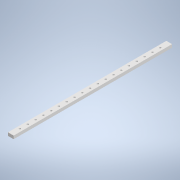
# Autodesk Inventor part: ServoArm
Saved by Autodesk Inventor 2020 (Build 240168000, 168)
## iProperties
Created: 2020-02-26
Part Number: ServoArm
Material: Generic
Document SubType Name: Modeling
Designer: shrey
Density: 1 g/cm^3
Appearance: Default
Author: shrey
Autodesk Inventor part; units mm, degrees
ref_plane "YZ Plane" through (0, 0, 0) normal (1, 0, 0) x (0, 1, 0)
ref_plane "XZ Plane" through (0, 0, 0) normal (0, 1, 0) x (-1, 0, 0)
ref_plane "XY Plane" through (0, 0, 0) normal (0, 0, 1) x (1, 0, 0)
sketch "Sketch1" plane through (0, 0, 0) normal (0, 1, 0) x (-1, 0, 0)
  line L0 (5.872, 162.6948) -> (-5.872, 162.6948)
  line L1 (-5.872, 162.6948) -> (-5.872, -162.6948)
  line L2 (-5.872, -162.6948) -> (5.872, -162.6948)
  line L3 (5.872, -162.6948) -> (5.872, 162.6948)
  line L4 (5.872, 162.6948) -> (-5.872, -162.6948) construction
  line L5 (-5.872, 162.6948) -> (5.872, -162.6948) construction
  circle A0 centre (0, 0) radius 1.85
  circle A1 centre (0, 16) radius 1.85
  circle A2 centre (0, 32) radius 1.85
  circle A3 centre (0, 48) radius 1.85
  circle A4 centre (0, 64) radius 1.85
  circle A5 centre (0, 80) radius 1.85
  circle A6 centre (0, 96) radius 1.85
  circle A7 centre (0, 112) radius 1.85
  circle A8 centre (0, 128) radius 1.85
  circle A9 centre (0, 144) radius 1.85
  circle A10 centre (0, -16) radius 1.85
  circle A11 centre (0, 0) radius 1.85
  circle A12 centre (0, 16) radius 1.85
  circle A13 centre (0, 32) radius 1.85
  circle A14 centre (0, 48) radius 1.85
  circle A15 centre (0, 64) radius 1.85
  circle A16 centre (0, 80) radius 1.85
  circle A17 centre (0, 96) radius 1.85
  circle A18 centre (0, 112) radius 1.85
  circle A19 centre (0, 128) radius 1.85
  circle A20 centre (0, -32) radius 1.85
  circle A21 centre (0, -16) radius 1.85
  circle A22 centre (0, 0) radius 1.85
  circle A23 centre (0, 16) radius 1.85
  circle A24 centre (0, 32) radius 1.85
  circle A25 centre (0, 48) radius 1.85
  circle A26 centre (0, 64) radius 1.85
  circle A27 centre (0, 80) radius 1.85
  circle A28 centre (0, 96) radius 1.85
  circle A29 centre (0, 112) radius 1.85
  circle A30 centre (0, -48) radius 1.85
  circle A31 centre (0, -32) radius 1.85
  circle A32 centre (0, -16) radius 1.85
  circle A33 centre (0, 0) radius 1.85
  circle A34 centre (0, 16) radius 1.85
  circle A35 centre (0, 32) radius 1.85
  circle A36 centre (0, 48) radius 1.85
  circle A37 centre (0, 64) radius 1.85
  circle A38 centre (0, 80) radius 1.85
  circle A39 centre (0, 96) radius 1.85
  circle A40 centre (0, -64) radius 1.85
  circle A41 centre (0, -48) radius 1.85
  circle A42 centre (0, -32) radius 1.85
  circle A43 centre (0, -16) radius 1.85
  circle A44 centre (0, 0) radius 1.85
  circle A45 centre (0, 16) radius 1.85
  circle A46 centre (0, 32) radius 1.85
  circle A47 centre (0, 48) radius 1.85
  circle A48 centre (0, 64) radius 1.85
  circle A49 centre (0, 80) radius 1.85
  circle A50 centre (0, -80) radius 1.85
  circle A51 centre (0, -64) radius 1.85
  circle A52 centre (0, -48) radius 1.85
  circle A53 centre (0, -32) radius 1.85
  circle A54 centre (0, -16) radius 1.85
  circle A55 centre (0, 0) radius 1.85
  circle A56 centre (0, 16) radius 1.85
  circle A57 centre (0, 32) radius 1.85
  circle A58 centre (0, 48) radius 1.85
  circle A59 centre (0, 64) radius 1.85
  circle A60 centre (0, -96) radius 1.85
  circle A61 centre (0, -80) radius 1.85
  circle A62 centre (0, -64) radius 1.85
  circle A63 centre (0, -48) radius 1.85
  circle A64 centre (0, -32) radius 1.85
  circle A65 centre (0, -16) radius 1.85
  circle A66 centre (0, 0) radius 1.85
  circle A67 centre (0, 16) radius 1.85
  circle A68 centre (0, 32) radius 1.85
  circle A69 centre (0, 48) radius 1.85
  circle A70 centre (0, -112) radius 1.85
  circle A71 centre (0, -96) radius 1.85
  circle A72 centre (0, -80) radius 1.85
  circle A73 centre (0, -64) radius 1.85
  circle A74 centre (0, -48) radius 1.85
  circle A75 centre (0, -32) radius 1.85
  circle A76 centre (0, -16) radius 1.85
  circle A77 centre (0, 0) radius 1.85
  circle A78 centre (0, 16) radius 1.85
  circle A79 centre (0, 32) radius 1.85
  circle A80 centre (0, -128) radius 1.85
  circle A81 centre (0, -112) radius 1.85
  circle A82 centre (0, -96) radius 1.85
  circle A83 centre (0, -80) radius 1.85
  circle A84 centre (0, -64) radius 1.85
  circle A85 centre (0, -48) radius 1.85
  circle A86 centre (0, -32) radius 1.85
  circle A87 centre (0, -16) radius 1.85
  circle A88 centre (0, 0) radius 1.85
  circle A89 centre (0, 16) radius 1.85
  circle A90 centre (0, -144) radius 1.85
  circle A91 centre (0, -128) radius 1.85
  circle A92 centre (0, -112) radius 1.85
  circle A93 centre (0, -96) radius 1.85
  circle A94 centre (0, -80) radius 1.85
  circle A95 centre (0, -64) radius 1.85
  circle A96 centre (0, -48) radius 1.85
  circle A97 centre (0, -32) radius 1.85
  circle A98 centre (0, -16) radius 1.85
  circle A99 centre (0, 0) radius 1.85
  dimension "d0" = 3.7
  dimension "d3" = 16
  dimension "d6" = 16
  constraints: 100 centre point, 12 end point, 2 midpoint, 2 parallel, 2 vertical, 1 coincident, 1 horizontal, 1 perpendicular, 198 other
  measures "d0" diameter of A0
  measures "d3" distance of A0.centre A1.centre
  measures "d6" distance of A0.centre A10.centre
extrude "Extrusion1" add sketch "Sketch1" along normal blind 6.35
body "Solid1"
